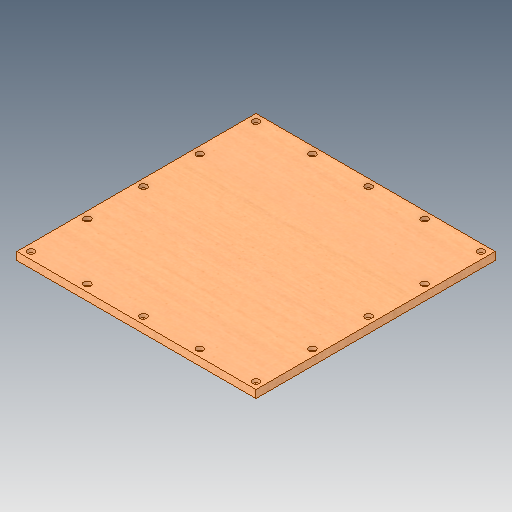
# Autodesk Inventor part: frontBackFace
Saved by Autodesk Inventor 2018.2 (Build 222227000, 227)
## iProperties
Created: 2016-04-01
Part Number: frontBackFace
Material: Wood (Cherry)
Document SubType Name: Modeling
Designer: sawai
Density: 0.63 g/cm^3
Appearance: Cherry - Natural Low Gloss
Author: sawai
Autodesk Inventor part; units mm, degrees
ref_plane "YZ Plane" through (0, 0, 0) normal (1, 0, 0) x (0, 1, 0)
ref_plane "XZ Plane" through (0, 0, 0) normal (0, 1, 0) x (-1, 0, 0)
ref_plane "XY Plane" through (0, 0, 0) normal (0, 0, 1) x (1, 0, 0)
sketch "Sketch1" plane through (0, 0, 0) normal (0, 1, 0) x (-1, 0, 0)
  line L0 (170, 170) -> (-170, 170)
  line L1 (-170, 170) -> (-170, -170)
  line L2 (-170, -170) -> (170, -170)
  line L3 (170, -170) -> (170, 170)
  line L4 (170, 170) -> (-170, -170) construction
  line L5 (-170, 170) -> (170, -170) construction
  point P0 (0, 0)
  dimension "d0" = 340
  dimension "d1" = 340
  constraints: 12 end point, 2 midpoint, 2 parallel, 1 horizontal, 1 perpendicular
  measures "d0" distance of L2.end L1.end
  measures "d1" distance between parallel lines of L0 L2
extrude "Extrusion1" add sketch "Sketch1" along normal blind 11.1125
sketch "Sketch2" plane through (0, 11.1125, 0) normal (0, 1, 0) x (1, 0, 0)
  line L0 (-170, -170) -> (170, -170) projected
  line L1 (170, -170) -> (170, 170) projected
  line L2 (170, 170) -> (-170, 170) projected
  line L3 (-170, 170) -> (-170, -170) projected
  point P0 (0, 0)
  point P1 (-160, -160)
  dimension "d4" = 10
  dimension "d5" = 10
  measures "d4" distance from line of L3 point (-160, -160)
  measures "d5" distance from line of L0 point (-160, -160)
hole "Hole1" at (-160, 11.1125, 160) direction (0, -1, 0) diameter 5.5 end through all counterbore diameter 10 counterbore depth 5 clearance for "Socket Head Cap Screw" size "M5" standard "Ansi Metric M Profile"
pattern_linear "Rectangular Pattern1" count 2 spacing 320 along (0, 0, -1) count 5 spacing 80 along (1, 0, 0) of "Hole1"
pattern_circular "Circular Pattern1" count 2 over 90 about axis through (0, -10, 0) along (0, 1, 0) of "Hole1", "Rectangular Pattern1"
equation "\"d2\" = facingThickness - facingGasketThickness"
equation "\"facingThickness\" = 12.7"
equation "\"facingGasketThickness\" = 1.5875"
body "Solid1"
